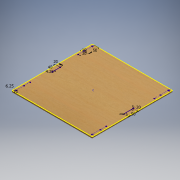
# Autodesk Inventor part: Floor
Saved by Autodesk Inventor 2019 (Build 230136000, 136)
## iProperties
Created: 2019-08-18
Part Number: Floor
Material: Generic
Document SubType Name: Modeling
Designer: Bruno
Density: 1 g/cm^3
Appearance: Default
Author: Bruno
Autodesk Inventor part; units mm, degrees
ref_plane "YZ Plane" through (0, 0, 0) normal (1, 0, 0) x (0, 1, 0)
ref_plane "XZ Plane" through (0, 0, 0) normal (0, 1, 0) x (-1, 0, 0)
ref_plane "XY Plane" through (0, 0, 0) normal (0, 0, 1) x (1, 0, 0)
sketch "Sketch1" plane through (0, 0, 0) normal (0, 1, 0) x (-1, 0, 0)
  line L0 (200, -200) -> (-200, -200)
  line L1 (-200, -200) -> (-200, 200)
  line L2 (-200, 200) -> (200, 200)
  line L3 (200, 200) -> (200, -200)
  line L4 (160, -160) -> (-160, -160)
  line L5 (-160, -160) -> (-160, 160)
  line L6 (-160, 160) -> (160, 160)
  line L7 (160, 160) -> (160, -160)
  line L8 (0, 42.2223) -> (0, -35.1237) construction
  line L9 (40.4991, 0) -> (-29.63, 0) construction
  point P0 (0, 0)
  dimension "d0" = 400
  dimension "d1" = 320
  dimension "d2" = 320
  dimension "d3" = 400
  constraints: 20 end point, 4 parallel, 3 horizontal, 2 perpendicular, 2 point on line, 1 vertical, 4 other
  measures "d0" distance of L0.start L0.end
  measures "d1" distance of L4.start L4.end
  measures "d2" distance of L6.end L4.start
  measures "d3" distance of L0.end L1.end
extrude "Extrusion1" add sketch "Sketch1" along normal blind 8 contours L0 L1 L2 L3 | L4 L5 L6 L7
sketch "Sketch3" plane through (0, 8, 0) normal (0, 1, 0) x (1, 0, 0)
  circle A0 centre (-190, 150) radius 2.5
  circle A1 centre (-190, 120) radius 2.5
  line L0 (-190, 120) -> (-190, 150) construction
  line L1 (-200, 200) -> (-200, -200) projected
  line L2 (-200, 150) -> (-190, 150) construction
  line L3 (-190, 150) -> (-190, 200) construction
  line L4 (200, 200) -> (-200, 200) projected
  circle A2 centre (-190, -120) radius 2.5
  circle A3 centre (-190, -150) radius 2.5
  circle A4 centre (190, -120) radius 2.5
  circle A5 centre (190, -150) radius 2.5
  circle A6 centre (190, 150) radius 2.5
  circle A7 centre (190, 120) radius 2.5
  line L5 (-190, -120) -> (-190, -150) construction
  line L6 (190, -150) -> (190, -120) construction
  line L7 (190, 120) -> (190, 150) construction
  line L8 (-190, -150) -> (-190, -200) construction
  line L9 (-200, -200) -> (200, -200) projected
  line L10 (-190, -150) -> (-200, -150) construction
  line L11 (190, -150) -> (190, -200) construction
  line L12 (200, -200) -> (200, 200) projected
  line L13 (190, -150) -> (200, -150) construction
  line L14 (190, 150) -> (200, 150) construction
  line L15 (190, 150) -> (190, 200) construction
  circle A8 centre (180, 25) radius 2.5
  circle A9 centre (180, -25) radius 2.5
  line L16 (180, 25) -> (180, -25)
  line L17 (0, 0) -> (0, 10.1722) construction
  line L18 (0, 0) -> (9.7219, 0) construction
  circle A10 centre (-180, -20) radius 2.125
  circle A11 centre (-180, 20) radius 2.125
  line L19 (-180, 20) -> (-180, -20)
  circle A12 centre (-190, -190) radius 3.125
  line L20 (-190, -190) -> (-190, -200) construction
  line L21 (-190, -190) -> (-200, -190) construction
  circle A13 centre (190, -190) radius 3.125
  circle A14 centre (190, 190) radius 3.125
  circle A15 centre (-190, 190) radius 3.125
  line L22 (190, -190) -> (200, -190) construction
  line L23 (190, -190) -> (190, -200) construction
  line L24 (190, 190) -> (200, 190)
  line L25 (190, 190) -> (190, 200) construction
  line L26 (-190, 190) -> (-200, 190) construction
  line L27 (-190, 190) -> (-190, 200) construction
  dimension "d6" = 5
  dimension "d7" = 30
  dimension "d8" = 50
  dimension "d9" = 10
  dimension "d12" = 50
  dimension "d13" = 5
  dimension "d14" = 5
  dimension "d15" = 20
  dimension "d16" = 4.25
  dimension "d17" = 40
  dimension "d18" = 20
  dimension "d19" = 6.25
  dimension "d20" = 10
  constraints: 48 end point, 16 centre point, 16 equal length, 16 point on line, 11 equal radius, 10 perpendicular, 10 vertical, 4 horizontal, 2 symmetric about line
  measures "d6" diameter of A0
  measures "d7" distance of L0.start L0.end
  measures "d8" distance of L0.end L3.end
  measures "d9" distance of L2.start L0.end
  measures "d12" distance of L16.end L16.start
  measures "d13" diameter of A8
  measures "d14" diameter of A9
  measures "d15" distance between parallel lines of L12 L16
  measures "d16" diameter of A10
  measures "d17" distance of L19.start L19.end
  measures "d18" distance between parallel lines of L1 L19
  measures "d19" diameter of A12
  measures "d20" distance of L20.start L20.end
extrude "Extrusion2" cut sketch "Sketch3" against normal through all contours A0 | A1 | A2 | A3 | A4 | A5 | A6 | A7 | A8 | A9 | A12 | A13 | A14 | A15
body "Solid1"
